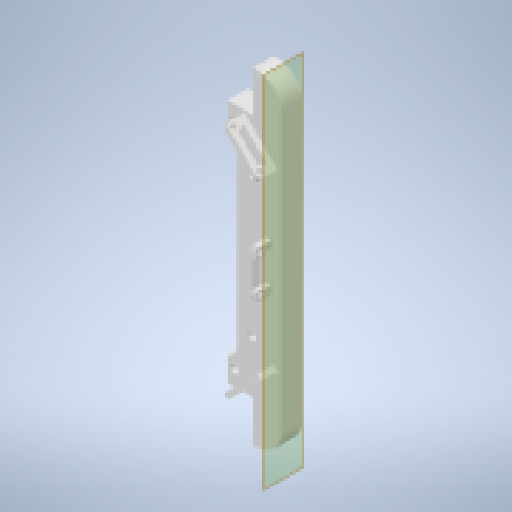
# Autodesk Inventor part: front_part_2
Saved by Autodesk Inventor 2023 (Build 270158000, 158)
## iProperties
Created: 2026-02-12
Part Number: front_part_2
Material: Типовые
Document SubType Name: Modeling
Designer: garin
Density: 1 g/cm^3
Appearance: По умолчанию
Author: garin
Autodesk Inventor part; units mm, degrees
ref_plane "YZ Plane" through (0, 0, 0) normal (1, 0, 0) x (0, 1, 0)
ref_plane "XZ Plane" through (0, 0, 0) normal (0, 1, 0) x (-1, 0, 0)
ref_plane "XY Plane" through (0, 0, 0) normal (0, 0, 1) x (1, 0, 0)
sketch "Эскиз1" plane through (0, 0, 0) normal (0, 0, 1) x (1, 0, 0)
  line L0 (0, 0) -> (90, 0)
  line L1 (90, 0) -> (90, 74.5)
  line L2 (123.0872, 0) -> (-138.0608, 0) construction
  line L3 (75, 74.5) -> (75, 65.5)
  line L4 (75, 65.5) -> (61.2, 65.5)
  line L5 (61.2, 65.5) -> (61.2, 52.2)
  line L6 (61.2, 52.2) -> (66.2, 52.2) construction
  line L7 (66.2, 52.2) -> (66.2, 47.2) construction
  line L8 (66.2, 47.2) -> (61.2, 47.2) construction
  line L9 (61.2, 47.2) -> (61.2, 52.2) construction
  arc A0 (66.2, 47.2) -> (61.2, 52.2) centre (61.2, 47.2) ccw
  line L10 (66.2, 47.2) -> (66.2, 0)
  line L11 (61.2, 52.2) -> (65.2, 52.2) construction
  line L12 (65.2, 52.2) -> (65.2, 57.2) construction
  line L13 (65.2, 57.2) -> (61.2, 57.2) construction
  line L14 (61.2, 57.2) -> (61.2, 52.2) construction
  circle A1 centre (65.2, 57.2) radius 2.1
  line L15 (75, 74.5) -> (75, 87.5)
  line L16 (75, 87.5) -> (77, 87.5)
  arc A2 (90, 74.5) -> (77, 87.5) centre (77, 74.5) ccw
  line L17 (90, 0) -> (90, -74.5)
  line L18 (75, -74.5) -> (75, -65.5)
  line L19 (75, -65.5) -> (61.2, -65.5)
  line L20 (61.2, -65.5) -> (61.2, -52.2)
  line L21 (61.2, -52.2) -> (66.2, -52.2) construction
  line L22 (66.2, -52.2) -> (66.2, -47.2) construction
  line L23 (66.2, -47.2) -> (61.2, -47.2) construction
  line L24 (61.2, -47.2) -> (61.2, -52.2) construction
  arc A3 (61.2, -52.2) -> (66.2, -47.2) centre (61.2, -47.2) ccw
  line L25 (66.2, -47.2) -> (66.2, 0)
  line L26 (61.2, -52.2) -> (65.2, -52.2) construction
  line L27 (65.2, -52.2) -> (65.2, -57.2) construction
  line L28 (65.2, -57.2) -> (61.2, -57.2) construction
  line L29 (61.2, -57.2) -> (61.2, -52.2) construction
  circle A4 centre (65.2, -57.2) radius 2.1
  line L30 (75, -74.5) -> (75, -87.5)
  line L31 (75, -87.5) -> (77, -87.5)
  arc A5 (77, -87.5) -> (90, -74.5) centre (77, -74.5) ccw
  circle A6 centre (81.192, 68.692) radius 2.1
  circle A7 centre (81.192, -68.692) radius 2.1
  line L32 (75, -65.5) -> (75, -37.341) construction
  line L33 (75, -37.341) -> (37.7624, -37.341) construction
  line L34 (66.2, -37.341) -> (74.621, -37.341) construction
  circle A8 centre (74.621, -37.341) radius 2.1
  circle A9 centre (74.621, 37.341) radius 2.1
  dimension "d0" = 90
  dimension "d1" = 74.5
  dimension "d2" = 15
  dimension "d3" = 9
  dimension "d4" = 13.8
  dimension "d5" = 13.3
  dimension "d6" = 5
  dimension "d7" = 5
  dimension "d8" = 4
  dimension "d9" = 5
  dimension "d10" = 4.2
  dimension "d13" = 13
  dimension "d14" = 2
  dimension "d49" = 4.2
  dimension "d83" = 28.159
  dimension "d84" = 8.421
  dimension "d85" = 4.2
  constraints: 70 end point, 18 symmetric about line, 10 centre point, 8 point on circle, 6 point on line, 5 perpendicular, 5 vertical, 4 horizontal, 4 parallel, 3 coincident, 2 tangent, 5 other
  measures "d0" distance of L0.start L0.end
  measures "d1" distance of L0.end L1.end
  measures "d2" distance of L1.end L3.start
  measures "d3" distance of L3.start L3.end
  measures "d4" distance of L3.end L4.end
  measures "d5" distance of L4.end L5.end
  measures "d6" distance of L7.end L8.end
  measures "d7" distance of L6.end L7.end
  measures "d8" distance of L13.end L12.end
  measures "d9" distance of L12.end L11.end
  measures "d10" diameter of A1
  measures "d13" distance of L3.start L15.end
  measures "d14" distance of L15.end L16.end
  measures "d49" diameter of A6
  measures "d83" distance of L19.start L32.end
  measures "d84" distance of L34.start L34.end
  measures "d85" diameter of A8
ref_plane "РабПлоскость1" through (-0.0152, -0.1454, 9) normal (0, 0, 1) x (0.9999948, 0.0032337, 0)
extrude "Выдавливание2" add sketch "Эскиз1" along normal blind 11 from surface at 9 contours L10 A0 L5 L4 L3 L15 L16 A2 L1 L0 | L0 L17 A5 L31 L30 L18 L19 L20 A3 L25 | A6 | A7 | A8 | A9
sketch "Эскиз2" plane through (61.2, -65.5, 20) normal (0, 0, 1) x (1, 0, 0)
  line L0 (0, 131) -> (13.8, 131) construction
  line L1 (0, 131) -> (7, 131) construction
  line L2 (7, 131) -> (7, 119) construction
  line L3 (7, 119) -> (0, 119) construction
  line L4 (0, 119) -> (0, 131) construction
  line L5 (7, 131) -> (7, 128) construction
  line L6 (26.9404, 112.3022) -> (24.8191, 110.1809)
  line L7 (24.8191, 110.1809) -> (7.1414, 127.8586)
  line L8 (24.8191, 110.1809) -> (49.8191, 110.1809) construction
  line L9 (7.1414, 127.8586) -> (9.2627, 129.9799)
  line L10 (9.2627, 129.9799) -> (26.9404, 112.3022)
  point P0 (-61.2, 65.5)
  dimension "d17" = 7
  dimension "d18" = 12
  dimension "d19" = 3
  dimension "d20" = 25.2
  dimension "d26" = 25
  dimension "d27" = 135
  constraints: 20 end point, 3 perpendicular, 2 horizontal, 2 parallel, 1 equal length, 1 point on line
  measures "d17" distance of L2.end L3.end
  measures "d18" distance of L1.end L2.end
  measures "d19" distance of L1.end L5.end
  measures "d20" distance of L5.end L6.end
  measures "d26" distance of L6.end L7.end
  measures "d27" angle of L8 L7
extrude "Выдавливание3" add sketch "Эскиз2" along normal blind 13
sketch "Эскиз4" plane through (70.4627, 64.4799, 20) normal (0.7071068, 0.7071068, 0) x (-0.7071068, 0.7071068, 0)
  line L0 (-25, 0) -> (-25, 13) construction
  line L1 (-25, 12.5) -> (-22.5, 12.5) construction
  line L2 (-25, 10) -> (-25, 12.5) construction
  circle A0 centre (-22.2, 10.5) radius 1.25
  circle A1 centre (-2.8, 10.5) radius 1.25
  line L3 (0, 13) -> (-25, 13) projected
  line L4 (-25, 12.5) -> (-21, 12.5) construction
  line L5 (-21, 12.5) -> (-21, 8.5) construction
  line L6 (-21, 8.5) -> (-25, 8.5) construction
  line L7 (-25, 8.5) -> (-25, 12.5) construction
  line L8 (-6.7296, 0) -> (-112.0886, 0) construction
  line L9 (-75.9554, 0) -> (-9.2045, 0) construction
  line L10 (-22.2, 10.5) -> (-22.2, 12) construction
  line L11 (0, 0) -> (-25, 0) projected
  line L12 (-22.2, 10.5) -> (-22.2, 13.5) construction
  line L13 (-25, 0) -> (0, 0) projected
  line L14 (-4, 0) -> (-21, 0)
  line L15 (-12.5, 13) -> (-14.5, 13) construction
  line L16 (-14.5, 13) -> (-10.5, 13) construction
  line L17 (-10.5, 13) -> (-10.5, 3)
  line L18 (-14.5, 3) -> (-14.5, 13)
  line L19 (-14.5, 3) -> (-10.5, 3)
  line L20 (-10.5, 13) -> (-14.5, 13)
  line L21 (0, 0) -> (0, 2.3) construction
  line L22 (0, 0) -> (0, 13) construction
  line L23 (0, 0) -> (2.3, 0) construction
  line L24 (0, 2.3) -> (-3.5, 2.3)
  line L25 (-3.5, 2.3) -> (-3.5, 7.4343)
  line L26 (-3.5, 7.4343) -> (0, 7.4343)
  line L27 (0, 7.4343) -> (0, 2.3)
  line L28 (-14.5, 13) -> (0, 13)
  line L29 (0, 13) -> (0, 2)
  line L30 (0, 2) -> (-14.5, 2)
  line L31 (-14.5, 2) -> (-14.5, 13)
  point P0 (4.2305, -20)
  point P1 (-22.5, 10.5)
  point P2 (-2.5, 10.5)
  point P3 (-2.8, 10.5)
  point P4 (-10.5, 13)
  point P5 (0, 7.4343)
  point P6 (-14.5, 3)
  dimension "d31" = 2.5
  dimension "d32" = 2.5
  dimension "d33" = 4
  dimension "d34" = 4
  dimension "d94" = 1.5
  dimension "d97" = 3
  dimension "d98" = 2
  dimension "d99" = 4
  dimension "d100" = 2.3
  dimension "d101" = 90
  dimension "d102" = 3.5
  dimension "d103" = 11
  dimension "d143" = 5.1343
  constraints: 50 end point, 8 horizontal, 7 parallel, 5 perpendicular, 3 coincident, 2 centre point, 2 point on line, 2 vertical, 1 collinear, 3 other
  measures "d31" diameter of A0
  measures "d32" diameter of A1
  measures "d33" distance of L5.end L6.end
  measures "d34" distance of L4.end L5.end
  measures "d94" distance of L10.start L10.end
  measures "d97" distance of L12.start L12.end
  measures "d98" distance of L15.start L15.end
  measures "d99" distance of L17.end L18.start
  measures "d100" distance of L11.start L21.end
  measures "d101" angle of L23 L21
  measures "d102" distance of L25.end L26.end
  measures "d103" distance of L28.end L29.end
  measures "d143" distance of L24.end L25.end
extrude "Выдавливание4" cut sketch "Эскиз4" against normal blind 3 contours A0 | A1
fillet "Сопряжение1" radius 2 2 edges at (87.0798, 45.7416, 33) (69.4021, 63.4192, 33)
sketch "Эскиз6" plane through (71.1698, 59.5302, 28.5) normal (-0.7071068, -0.7071068, 0) x (-0.7071068, 0.7071068, 0)
  line L0 (-1, 0.0575) -> (-16, 0.0575)
  line L1 (-16, 0.0575) -> (-16, -4)
  line L2 (-16, -4) -> (-1, -4)
  line L3 (-1, -4) -> (-1, 0.0575)
  point P0 (8.2305, 28.5)
  dimension "d42" = 15
  constraints: 8 end point, 2 parallel, 1 horizontal, 1 perpendicular
  measures "d42" distance of L2.end L1.end
extrude "Выдавливание6" cut sketch "Эскиз1" along normal blind 8 from surface at 9 contours A6 | A7
sketch "Эскиз8" plane through (61.2, 65.5, 20) normal (0, 0, 1) x (1, 0, 0)
  line L0 (28.8, 9) -> (28.8, -140) projected
  line L1 (23.8, -53) -> (20.8, -53)
  line L2 (20.8, -53) -> (20.8, -78)
  line L3 (20.8, -78) -> (23.8, -78)
  line L4 (23.8, -78) -> (23.8, -53)
  point P0 (-61.2, -65.5)
  point P1 (28.8, -63)
  point P2 (28.8, -65.5)
  dimension "d54" = 3
  dimension "d55" = 25
  constraints: 8 end point, 2 parallel, 1 horizontal, 1 midpoint, 1 perpendicular, 1 point on line
  measures "d54" distance of L3.end L2.end
  measures "d55" distance of L2.end L1.end
extrude "Выдавливание7" add sketch "Эскиз8" along normal blind 13
sketch "Эскиз10" plane through (85, -12.5, 20) normal (1, 0, 0) x (0, 0, -1)
  line L0 (-13, 0) -> (-10.5, 0) construction
  line L1 (-10.5, 0) -> (-10.5, 2.8) construction
  line L2 (-10.5, 2.8) -> (-13, 2.8) construction
  line L3 (-13, 2.8) -> (-13, 0) construction
  circle A0 centre (-10.5, 2.8) radius 1.25
  line L4 (-10.5, 2.8) -> (-10.5, 22.2) construction
  circle A1 centre (-10.5, 22.2) radius 1.25
  line L5 (-13, 0) -> (-9, 0) construction
  line L6 (-9, 0) -> (-9, 4) construction
  line L7 (-9, 4) -> (-13, 4) construction
  line L8 (-13, 4) -> (-13, 0) construction
  line L9 (-13, 0) -> (-13, 25) construction
  line L10 (-13, 0) -> (-13, 5) construction
  line L11 (-13, 20) -> (-13, 5)
  line L12 (0, 87) -> (0, -62) projected
  line L13 (0, 25) -> (-2, 25)
  line L14 (-2, 25) -> (-2, 10.5)
  line L15 (-2, 10.5) -> (0, 10.5)
  line L16 (0, 10.5) -> (0, 25)
  line L17 (-2, 10.5) -> (-13, 10.5)
  line L18 (-13, 10.5) -> (-3, 10.5)
  line L19 (-3, 10.5) -> (-3, 14.5)
  line L20 (-3, 14.5) -> (-13, 14.5)
  line L21 (-13, 14.5) -> (-13, 10.5)
  line L22 (-2, 25) -> (-2.3, 25)
  line L23 (0, 25) -> (-13, 25) projected
  line L24 (-2.3, 25) -> (-7.434, 25)
  line L25 (-7.434, 25) -> (-7.434, 21.5)
  line L26 (-7.434, 21.5) -> (-2.3, 21.5)
  line L27 (-2.3, 21.5) -> (-2.3, 25)
  line L28 (-13, 25) -> (-13, 0) projected
  line L29 (-13, 10.5) -> (-13, 25)
  line L30 (-13, 25) -> (-2, 25)
  line L31 (0, 25) -> (-13, 25)
  line L32 (-13, 25) -> (-13, 10.5)
  line L33 (-13, 10.5) -> (0, 10.5)
  line L34 (0, 10.5) -> (0, 25)
  point P0 (20, 12.5)
  dimension "d67" = 2.5
  dimension "d68" = 2.8
  dimension "d69" = 2.5
  dimension "d70" = 19.4
  dimension "d71" = 2.5
  dimension "d72" = 4
  dimension "d73" = 4
  dimension "d76" = 5
  dimension "d144" = 2
  dimension "d145" = 14.5
  dimension "d146" = 10
  dimension "d147" = 4
  dimension "d148" = 0.3
  dimension "d149" = 5.134
  dimension "d150" = 3.5
  constraints: 62 end point, 12 parallel, 8 perpendicular, 6 horizontal, 4 point on line, 2 centre point, 2 coincident, 2 vertical
  measures "d67" distance of L2.end L1.end
  measures "d68" distance of L1.end L0.end
  measures "d69" diameter of A0
  measures "d70" distance of L4.start L4.end
  measures "d71" diameter of A1
  measures "d72" distance of L7.end L6.end
  measures "d73" distance of L6.end L5.end
  measures "d76" distance of L0.start L10.end
  measures "d144" distance of L15.end L14.end
  measures "d145" distance of L14.end L13.end
  measures "d146" distance of L20.end L19.end
  measures "d147" distance of L19.end L18.end
  measures "d148" distance of L13.end L22.end
  measures "d149" distance of L26.end L25.end
  measures "d150" distance of L25.end L24.end
extrude "Выдавливание8" cut sketch "Эскиз10" against normal blind 3 contours A0 | A1
extrude "Выдавливание9" [suppressed]
fillet "Сопряжение2" radius 2 2 edges at (83.5, 12.5, 33) (83.5, -12.5, 33)
ref_plane "РабПлоскость2" through (90, -37.25, 9) normal (-1, 0, 0) x (0, -1, 0)
extrude "Выдавливание10" cut sketch "Эскиз1" against normal blind 7 from surface at 20 contours A8 | A9
extrude "Выдавливание11" cut sketch "Эскиз4" against normal blind 3 contours L17 L19 L18 L3 | L27 L24 L25 L26
extrude "Выдавливание12" cut sketch "Эскиз4" against normal blind 1 contours L29 L26 L25 L24 L30 L31 L19 L17 L3
mirror "Зеркальное отражение6" about plane through (0, 0, 0) normal (0, 1, 0) of "Выдавливание3", "Сопряжение1", "Выдавливание4"
sketch "Эскиз14" plane through (70.4627, -64.4799, 31) normal (0.7071068, -0.7071068, 0) x (-0.7071068, -0.7071068, 0)
  line L0 (-25, 11) -> (-25, 0) construction
  line L1 (-25, 11) -> (-10.5, 11) construction
  line L2 (-10.5, 11) -> (-10.5, 8.7) construction
  line L3 (-10.5, 8.7) -> (-25, 8.7) construction
  line L4 (-25, 8.7) -> (-25, 11) construction
  line L5 (-2, -2) -> (-23, -2) projected
  line L6 (-10.5, -2) -> (-25, -2)
  line L7 (-25, -2) -> (-25, 9)
  line L8 (-25, 9) -> (-10.5, 9)
  line L9 (-10.5, 9) -> (-10.5, -2)
  line L10 (-25, 8.7) -> (-21.5, 8.7)
  line L11 (-21.5, 8.7) -> (-21.5, 3.566)
  line L12 (-21.5, 3.566) -> (-25, 3.566)
  line L13 (-25, 3.566) -> (-25, 8.7)
  line L14 (-10.5, -2) -> (-14.5, -2)
  line L15 (-14.5, -2) -> (-14.5, 8)
  line L16 (-14.5, 8) -> (-10.5, 8)
  line L17 (-10.5, 8) -> (-10.5, -2)
  point P0 (4.2305, 31)
  point P1 (-10.5, 8)
  point P2 (-25, 3.566)
  dimension "d131" = 14.5
  dimension "d132" = 2.3
  dimension "d133" = 14.5
  dimension "d134" = 11
  dimension "d135" = 3.5
  dimension "d136" = 5.134
  dimension "d137" = 4
  dimension "d138" = 10
  constraints: 32 end point, 8 parallel, 4 horizontal, 4 perpendicular, 1 point on line
  measures "d131" distance of L2.end L3.end
  measures "d132" distance of L1.end L2.end
  measures "d133" distance of L7.end L8.end
  measures "d134" distance of L6.end L7.end
  measures "d135" distance of L11.end L12.end
  measures "d136" distance of L10.end L11.end
  measures "d137" distance of L15.end L16.end
  measures "d138" distance of L14.end L15.end
extrude "Выдавливание13" cut sketch "Эскиз14" against normal blind 3 contours L5 L15 L16 L9 | L7 L10 L11 L12
extrude "Выдавливание14" cut sketch "Эскиз14" against normal blind 1 contours L5 L6 L7 L12 L11 L10 L8 L9 L16 L15
sketch "Эскиз15" plane through (85, -12.5, 20) normal (1, 0, 0) x (0, 0, -1)
  line L0 (-10.5, 2.8) -> (-10.5, 22.2) construction
  circle A0 centre (-10.5, 22.2) radius 1.25
  line L1 (-13, 0) -> (-13, 25) construction
  line L2 (0, 87) -> (0, -62)
  line L3 (0, 25) -> (-2, 25)
  line L4 (-2, 25) -> (-2, 10.5)
  line L5 (-2, 10.5) -> (0, 10.5)
  line L6 (0, 10.5) -> (0, 25)
  line L7 (-2, 10.5) -> (-13, 10.5)
  line L8 (-13, 10.5) -> (-3, 10.5)
  line L9 (-3, 10.5) -> (-3, 14.5)
  line L10 (-3, 14.5) -> (-13, 14.5)
  line L11 (-13, 14.5) -> (-13, 10.5)
  line L12 (-2, 25) -> (-2.3, 25)
  line L13 (0, 25) -> (-13, 25)
  line L14 (-2.3, 25) -> (-7.434, 25)
  line L15 (-7.434, 25) -> (-7.434, 21.5)
  line L16 (-7.434, 21.5) -> (-2.3, 21.5)
  line L17 (-2.3, 21.5) -> (-2.3, 25)
  line L18 (-13, 10.5) -> (-13, 25)
  line L19 (-13, 25) -> (-2, 25)
  line L20 (0, 25) -> (-13, 25)
  line L21 (-13, 25) -> (-13, 10.5)
  line L22 (-13, 10.5) -> (0, 10.5)
  line L23 (0, 10.5) -> (0, 25)
  point P0 (20, 12.5)
  point P1 (-13, 2.8)
  point P2 (-13, 4)
  point P3 (-13, 5)
  point P4 (-13, 20)
  point P5 (-2.3, 25)
  point P6 (-7.434, 25)
  dimension "d151" = 19.4
  dimension "d152" = 2.5
  dimension "d153" = 5
  dimension "d154" = 2
  dimension "d155" = 14.5
  dimension "d156" = 10
  dimension "d157" = 4
  dimension "d158" = 0.3
  dimension "d159" = 5.134
  dimension "d160" = 3.5
  constraints: 48 end point, 8 parallel, 6 perpendicular, 4 horizontal, 3 point on line, 2 vertical, 1 centre point, 1 coincident
  measures "d151" distance of L0.start L0.end
  measures "d152" diameter of A0
  measures "d153" distance of L1.start point (-13, 5)
  measures "d154" distance of L6.start L7.start
  measures "d155" distance of L7.start L4.start
  measures "d156" distance of L10.end L10.start
  measures "d157" distance of L10.start L8.end
  measures "d158" distance of L4.start L12.end
  measures "d159" distance of L16.end L16.start
  measures "d160" distance of L16.start L15.start
extrude "Выдавливание15" cut sketch "Эскиз10" against normal blind 1 contours L28 L23 L25 L26 L27 L22 L14 L17 L19 L20 L11 | L20 L19 L17 L11 | L23 L27 L26 L25
extrude "Выдавливание16" cut sketch "Эскиз15" against normal blind 3 contours L17 L16 L15 L13 | L7 L11 L10 L9
